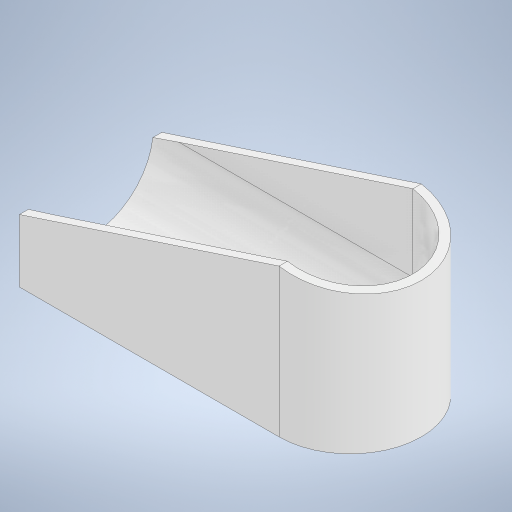
# Autodesk Inventor part: Receptor pequeno
Saved by Autodesk Inventor 2024 (Build 280153000, 153)
## iProperties
Created: 2023-05-09
Part Number: Receptor pequeno
Material: Plástico PET
Document SubType Name: Modeling
Designer: jpjoa
Density: 1.541 g/cm^3
Appearance: Branco
Author: jpjoa
Autodesk Inventor part; units mm, degrees
ref_plane "YZ Plane" through (0, 0, 0) normal (1, 0, 0) x (0, 1, 0)
ref_plane "XZ Plane" through (0, 0, 0) normal (0, 1, 0) x (-1, 0, 0)
ref_plane "XY Plane" through (0, 0, 0) normal (0, 0, 1) x (1, 0, 0)
sketch "Esboço1" plane through (0, 0, 0) normal (0, 1, 0) x (-1, 0, 0)
  line L0 (-1.2, -1.2) -> (-37.2, -1.2)
  line L1 (-1.2, -19.2) -> (-1.2, -1.2)
  arc A0 (-37.2, -1.2) -> (-37.2, -19.2) centre (-37.2, -10.2) ccw
  line L2 (-1.2, -19.2) -> (-37.2, -19.2)
  line L3 (-37.2, -20.4) -> (0, -20.4)
  line L4 (0, -20.4) -> (0, 0)
  line L5 (0, 0) -> (-37.2, 0)
  arc A1 (-37.2, 0) -> (-37.2, -20.4) centre (-37.2, -10.2) ccw
  line L6 (-1.2, -1.2) -> (0, -1.2)
  line L7 (-1.2, -19.2) -> (0, -19.2)
  point P0 (-1.2, -10.2)
  dimension "d0" = 18
  dimension "d3" = 18
  dimension "d5" = 36
  dimension "d6" = 1.2
  constraints: 16 end point, 4 point on circle, 3 horizontal alignment, 2 centre point, 2 coincident, 2 horizontal, 2 perpendicular, 2 point on line, 1 midpoint, 1 vertical alignment, 3 other
  measures "d0" distance of L1.start L0.start
  measures "d3" diameter of A0
  measures "d5" distance from line of L1 A0.centre
  measures "d6" radial gap between concentric circles of A0 A1
extrude "Extrusão1" add sketch "Esboço1" against normal blind 1.2
extrude "Extrusão2" add sketch "Esboço1" along normal blind 20 contours L0 A0 L2 L7 L4 L3 A1 L5 L6
fillet "Arredondamento1" radius 9 3 edges at (46.2, 0, -10.2) (18.6, 0, -1.2) (18.6, 0, -19.2)
sketch "Esboço2" plane through (0, -1.2, 0) normal (0, 0, 1) x (1, 0, 0)
  line L0 (37.2, 21.2) -> (46.2, 21.2) projected
  line L1 (37.2, 0) -> (0, 0) projected
  line L2 (37.2, 1.2) -> (37.2, 21.2) projected
  line L3 (0, 21.2) -> (0, 0) projected
  line L4 (47.4, 21.2) -> (37.2, 21.2) projected
  line L5 (0, 9) -> (37.2, 21.2)
  line L6 (37.2, 21.2) -> (0, 21.2)
  line L7 (0, 21.2) -> (37.2, 21.2) projected
  line L8 (37.2, 21.2) -> (47.4, 19.4015)
  line L9 (47.4, 21.2) -> (47.4, 0) projected
  line L10 (37.2, 21.2) -> (47.5574, 21.2) construction
  line L11 (47.4, 19.4015) -> (47.4, 21.2)
  line L12 (47.4, 21.2) -> (47.4, 0) projected
  line L13 (37.2, 21.2) -> (47.4, 21.2)
  line L14 (0, 9) -> (0, 21.2)
  point P0 (0, 1.2)
  point P1 (0, 10.6)
  point P2 (0, 10.6)
  dimension "d13" = 9
  dimension "d16" = 10
  constraints: 14 end point, 3 collinear, 2 midpoint, 1 equal length, 1 horizontal, 1 perpendicular, 1 point on line, 1 vertical alignment
  measures "d13" distance from line of L1 L5.start
  measures "d16" angle of L8 L10
extrude "Extrusão3" cut sketch "Esboço2" against normal up to surface (20.4 mm away)
equation "\"d0\" = Diâmetro_esfera"
equation "\"d3\" = Diâmetro_esfera"
equation "\"d5\" = 2 * Diâmetro_esfera"
equation "\"d6\" = Margem"
equation "\"d7\" = Margem"
equation "\"d11\" = 0.5 * Diâmetro_esfera"
equation "\"d13\" = 0.5 * Diâmetro_esfera"
equation "\"Diâmetro_esfera\" = 18"
equation "\"Filamento\" = 0.4"
equation "\"Margem\" = 3 * Filamento"
equation "\"Parafuso\" = 3"
